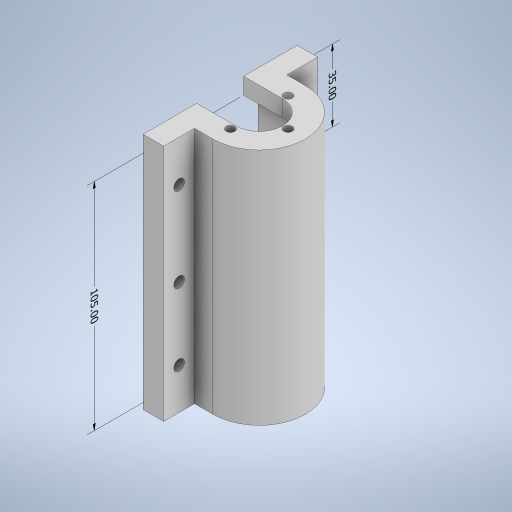
# Autodesk Inventor part: motor-fastening
Saved by Autodesk Inventor 2023 (Build 270158000, 158)
## iProperties
Created: 2024-03-10
Part Number: motor-fastening
Material: Genérico
Document SubType Name: Modeling
Designer: inigo
Density: 1 g/cm^3
Appearance: Valor por defecto
Author: inigo
Autodesk Inventor part; units mm, degrees
ref_plane "YZ Plane" through (0, 0, 0) normal (1, 0, 0) x (0, 1, 0)
ref_plane "XZ Plane" through (0, 0, 0) normal (0, 1, 0) x (-1, 0, 0)
ref_plane "XY Plane" through (0, 0, 0) normal (0, 0, 1) x (1, 0, 0)
sketch "Boceto1" plane through (0, 0, 0) normal (0, 1, 0) x (-1, 0, 0)
  circle A0 centre (0, 0) radius 14
  circle A1 centre (0, 14) radius 2.1
  circle A2 centre (0, 0) radius 11
  line L0 (0, 18.1) -> (19, 18.1)
  arc A3 (0, 18.1) -> (-18.1, 0) centre (0, 0) ccw
  line L1 (0, 0) -> (5.461, 0)
  arc A4 (0, 11.4) -> (-11.4, 0) centre (0, 0) ccw
  line L2 (0, 11.4) -> (19, 11.4)
  circle A5 centre (0, -14) radius 2.1
  line L3 (0, -18.1) -> (19, -18.1)
  arc A6 (-18.1, 0) -> (0, -18.1) centre (0, 0) ccw
  arc A7 (-11.4, 0) -> (0, -11.4) centre (0, 0) ccw
  line L4 (0, -11.4) -> (19, -11.4)
  circle A8 centre (-14, 0) radius 2.1
  circle A9 centre (0, 0) radius 19
  line L5 (19, 11.4) -> (19, 18.1)
  line L6 (19, -11.4) -> (19, -18.1)
  point P0 (8.1265, 11.4)
  point P1 (8.1265, 18.1)
  point P2 (8.1265, -11.4)
  point P3 (8.1265, -18.1)
  dimension "d0" = 28
  dimension "d1" = 4.2
  dimension "d3" = 22
  dimension "d12" = 11.4
  dimension "d18" = 4.2
  dimension "d19" = 38
  constraints: 14 end point, 12 point on circle, 10 centre point, 4 coincident, 4 point on line, 4 symmetric about line, 3 horizontal, 2 tangent, 2 vertical, 3 other
  measures "d0" diameter of A0
  measures "d1" diameter of A1
  measures "d3" diameter of A2
  measures "d12" radius of A4
  measures "d18" diameter of A8
  measures "d19" diameter of A9
extrude "Extrusión1" add sketch "Boceto1" along normal blind 8 contours L2 A4 A7 L4 A0 A5 A8 A1 | A0 A1 A8 A5 L4 A9 L3 A6 A3 L0 L2 | A9 L0 L5 L2 | L4 L6 L3 A9
sketch "Boceto2" plane through (0, 0, 0) normal (0, -1, 0) x (1, 0, 0)
  arc A0 (0, -18.5) -> (0, 18.5) centre (0, 0) ccw
  line L0 (0, 18.5) -> (-19, 18.5)
  line L1 (0, 22.5) -> (-19, 22.5)
  line L2 (0, -18.5) -> (-19, -18.5)
  line L3 (0, -22.5) -> (-19, -22.5)
  arc A1 (0, -22.5) -> (0, 22.5) centre (0, 0) ccw
  line L4 (-19, 18.1) -> (0, 18.1) projected
  line L5 (-19, 18.1) -> (-19, 18.5)
  line L6 (-19, -18.1) -> (-19, -11.4) projected
  line L7 (-19, -18.1) -> (-19, -18.5)
  line L8 (-19, 22.5) -> (-19, 24.19)
  line L9 (-19, 18.5) -> (-19, 22.5)
  line L10 (-19, -18.5) -> (-19, -22.5)
  line L11 (-19, -22.5) -> (-19, -24.4563)
  point P0 (-8.1265, 18.5)
  point P1 (-8.1265, 18.1)
  point P2 (-8.1265, 22.5)
  point P3 (-8.1265, -18.5)
  point P4 (-8.1265, -22.5)
  dimension "d14" = 37
  constraints: 20 end point, 6 vertical, 5 point on line, 4 horizontal, 4 point on circle, 3 tangent, 2 centre point, 1 coincident
  measures "d14" diameter of A0
extrude "Extrusión2" add sketch "Boceto2" along normal blind 35
sketch "Boceto3" plane through (0, 0, 0) normal (0, 1, 0) x (1, 0, 0)
  line L0 (0, 18.1) -> (-19, 18.1) projected
  line L1 (-8.1265, 18.1) -> (0, 18.1)
  line L2 (-8.1265, -11.4) -> (-8.1265, -18.1) projected
  arc A0 (0, -18.1) -> (0, 18.1) centre (0, 0) ccw projected
  line L3 (-8.1265, -18.1) -> (0, -18.1)
  arc A1 (-8.1265, -16.1731) -> (0, 18.1) centre (0, 0) ccw
  line L4 (-8.1265, -22.5) -> (-8.1265, -18.5) projected
  line L5 (-8.1265, -18.1) -> (-8.1265, -22.5)
  line L6 (-8.1265, -22.5) -> (0, -22.5)
  line L7 (-19, 22.5) -> (0, 22.5) projected
  line L8 (-8.1265, 22.5) -> (0, 22.5)
  arc A2 (0, -22.5) -> (0, 22.5) centre (0, 0) ccw
  line L9 (-19, -22.5) -> (-19, 22.5)
  line L10 (-8.1265, 18.1) -> (-19, 18.1)
  line L11 (-19, 22.5) -> (-8.1265, 22.5)
  line L12 (0, -22.5) -> (-19, -22.5) projected
  line L13 (-8.1265, -22.5) -> (-19, -22.5)
  line L14 (-19, -11.4) -> (-19, -18.1) projected
  line L15 (-19, -22.5) -> (-19, -18.1)
  line L16 (-19, -18.1) -> (-8.1265, -18.1)
  line L17 (-19, -18.1) -> (0, -18.1) projected
  constraints: 22 end point, 7 collinear, 4 point on circle, 3 perpendicular, 2 centre point, 2 coincident, 1 horizontal, 1 point on line, 1 tangent
extrude "Extrusión3" add sketch "Boceto3" along normal blind 8 contours L0 L9 L7 A2 L6 L4 L5 L3 A0 | L5 L4 L12 L9 L16
sketch "Boceto4" plane through (0, -35, 0) normal (0, -1, 0) x (1, 0, 0)
  line L0 (0, 19.5) -> (-19, 19.5)
  line L1 (-19, 22.5) -> (-19, 18.5) projected
  line L2 (-19, 22.5) -> (-19, 19.5)
  line L3 (0, -19.5) -> (-19, -19.5)
  line L4 (-19, -22.5) -> (-19, -11.4) projected
  line L5 (-19, -22.5) -> (-19, -19.5)
  line L6 (-19, -22.5) -> (0, -22.5) projected
  line L7 (-19, -22.5) -> (0, -22.5)
  arc A0 (0, -22.5) -> (0, 22.5) centre (0, 0) ccw projected
  line L8 (-19, 22.5) -> (0, 22.5) projected
  line L9 (0, 22.5) -> (-19, 22.5)
  arc A1 (0, -19.5) -> (0, 19.5) centre (0, 0) ccw
  arc A2 (0, -22.5) -> (0, 22.5) centre (0, 0) ccw
  constraints: 12 end point, 4 point on circle, 3 perpendicular, 2 centre point, 2 coincident, 2 collinear, 2 point on line, 1 horizontal
extrude "Extrusión4" add sketch "Boceto4" along normal blind 70
sketch "Boceto5" plane through (0, -105, 0) normal (0, -1, 0) x (1, 0, 0)
  line L0 (0, -22.5) -> (-19, -22.5) projected
  line L1 (0, -22.5) -> (-19, -22.5)
  line L2 (-19, -22.5) -> (-19, -11.4) projected
  line L3 (-19, 22.5) -> (0, 22.5) projected
  line L4 (-19, -22.5) -> (-19, 22.5)
  arc A0 (0, -22.5) -> (0, 22.5) centre (0, 0) ccw
  constraints: 5 end point, 2 point on circle, 1 centre point, 1 coincident, 1 collinear, 1 perpendicular
extrude "Extrusión5" add sketch "Boceto5" along normal blind 3
sketch "Boceto6" plane through (-19, 0, 11.4) normal (-1, 0, 0) x (0, 0, 1)
  line L0 (-33.9, 8) -> (-48.9, 8)
  line L1 (-48.9, 8) -> (-48.9, -32)
  line L2 (-48.9, -108) -> (-33.9, -108)
  line L3 (-33.9, -108) -> (-33.9, 8)
  circle A0 centre (-41.4, -53) radius 2.6
  line L4 (-48.9, -32) -> (-48.9, -108)
  line L5 (-48.9, -12) -> (-33.9, -12)
  circle A1 centre (-41.4, -12) radius 2.6
  line L6 (-11.4, 2) -> (-11.4, -20.5205)
  line L7 (-48.9, -50) -> (-33.9, -50)
  line L8 (-33.9, 8) -> (-33.9, -108) projected
  circle A2 centre (-41.4, -88) radius 2.6
  line L9 (11.1, 8) -> (26.1, 8)
  line L10 (26.1, 8) -> (26.1, -32)
  line L11 (26.1, -108) -> (11.1, -108)
  line L12 (11.1, -108) -> (11.1, 8)
  circle A3 centre (18.6, -53) radius 2.6
  line L13 (26.1, -32) -> (26.1, -108)
  line L14 (26.1, -12) -> (11.1, -12)
  circle A4 centre (18.6, -12) radius 2.6
  line L15 (26.1, -50) -> (11.1, -50)
  line L16 (11.1, 8) -> (11.1, -108)
  circle A5 centre (18.6, -88) radius 2.6
  point P0 (-11.4, 0)
  point P1 (11.1, 8)
  dimension "d25" = 15
  dimension "d26" = 5.2
  dimension "d27" = 5.2
  dimension "d28" = 20
  constraints: 32 end point, 13 symmetric about line, 6 centre point, 4 point on line, 3 midpoint, 3 parallel, 2 horizontal, 2 perpendicular, 1 vertical, 4 other
  measures "d25" distance of L2.end L2.start
  measures "d26" diameter of A0
  measures "d27" diameter of A1
  measures "d28" distance between parallel lines of L0 L5
extrude "Extrusión6" add sketch "Boceto6" against normal blind 10 contours L3 L5 A1 L1 L0 | L3 L7 L4 L1 L5 A1 | L3 L2 L4 L7 | L9 L10 L14 A4 L12 | L14 A4 L10 L13 L15 L12 | L15 L13 L11 L12
